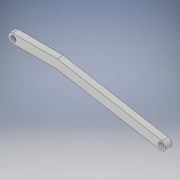
# Autodesk Inventor part: Ladebügel
Saved by Autodesk Inventor 2019 (Build 230136000, 136)
## iProperties
Created: 2022-03-16
Part Number: Ladebügel
Material: Generic
Document SubType Name: Modeling
Designer: Lukas
Density: 1 g/cm^3
Appearance: Default
Author: Lukas
Autodesk Inventor part; units mm, degrees
ref_plane "YZ Plane" through (0, 0, 0) normal (1, 0, 0) x (0, 1, 0)
ref_plane "XZ Plane" through (0, 0, 0) normal (0, 1, 0) x (-1, 0, 0)
ref_plane "XY Plane" through (0, 0, 0) normal (0, 0, 1) x (1, 0, 0)
sketch "Sketch1" plane through (0, 0, 0) normal (0, 0, 1) x (1, 0, 0)
  line L0 (0, 0) -> (-27.0626, 0)
  line L1 (0, 0) -> (60.6273, -10.6902)
  line L2 (60.6273, -10.6902) -> (61.4955, -5.7662)
  line L3 (61.4955, -5.7662) -> (0.4374, 5)
  line L4 (0.4374, 5) -> (-27.0626, 5)
  line L5 (-27.0626, 5) -> (-27.0626, 0)
  circle A0 centre (-24.0626, 2.5) radius 1.5
  circle A1 centre (58.5994, -7.7941) radius 1.6
  point P0 (-27.0626, 2.5)
  dimension "d0" = 5
  dimension "d1" = 5
  dimension "d2" = 27.5
  dimension "d3" = 62
  dimension "d4" = 170
  dimension "d5" = 2.5
  dimension "d6" = 2.5
  dimension "d7" = 3.2
  dimension "d8" = 3
  dimension "d9" = 3
  constraints: 12 end point, 2 centre point, 2 parallel, 2 perpendicular, 1 horizontal, 1 horizontal alignment, 1 midpoint
  measures "d0" distance between parallel lines of L4 L0
  measures "d1" distance between parallel lines of L3 L1
  measures "d2" distance of L3.end L4.end
  measures "d3" distance of L2.end L3.end
  measures "d4" angle of L0 L1
  measures "d5" distance from line of L1 A1.centre
  measures "d6" distance from line of L2 A1.centre
  measures "d7" diameter of A1
  measures "d8" distance from line of L5 A0.centre
  measures "d9" diameter of A0
extrude "Extrusion1" add sketch "Sketch1" along normal mid plane 3.5
fillet "Fillet1" radius 2.5 4 edges at (61.4955, -5.7662, 0) (60.6273, -10.6902, 0) (-27.0626, 0, 0) (-27.0626, 5, 0)
equation "\"d1\" = d0"
equation "\"d5\" = 0.5 * d1"
equation "\"d6\" = d5"
body "Solid1"
